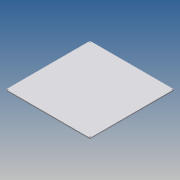
# Autodesk Inventor part: Aluplatte_5mm
Saved by Autodesk Inventor 2015 SP1 (Build 190203100, 203)
## iProperties
Created: 2015-03-05
Part Number: Aluplatte_5mm
Material: Aluminium 6061
Document SubType Name: Modeling
Designer: Marc
Mass: 1652.69 g
Surface Area: 2521.57 cm^2
Volume: 612.107 cm^3
Density: 2.7 g/cm^3
Appearance: Aluminium - flach
Author: Marc
Autodesk Inventor part; units mm, degrees
ref_plane "YZ Plane" through (0, 0, 0) normal (1, 0, 0) x (0, 1, 0)
ref_plane "XZ Plane" through (0, 0, 0) normal (0, 1, 0) x (-1, 0, 0)
ref_plane "XY Plane" through (0, 0, 0) normal (0, 0, 1) x (1, 0, 0)
sketch "Skizze1" plane through (0, 0, 0) normal (0, 0, 1) x (1, 0, 0)
  line L0 (0, -266) -> (0, 266) projected
  line L1 (-266, 0) -> (266, 0) projected
  line L2 (-190, -190) -> (190, -190)
  line L3 (190, -190) -> (190, 190)
  line L4 (190, 190) -> (-190, 190)
  line L5 (-190, 190) -> (-190, -190)
  line L6 (-190, -190) -> (190, 190) construction
  line L7 (190, -190) -> (-190, 190) construction
  point P0 (0, 0)
  dimension "d0" = 380
  dimension "d1" = 380
  constraints: 12 end point, 2 midpoint, 2 parallel, 1 horizontal, 1 perpendicular
  measures "d0" distance of L4.end L3.end
  measures "d1" distance of L3.end L2.end
extrude "Extrusion1" add sketch "Skizze1" along normal blind 5
sketch "Skizze2" plane through (0, 0, 5) normal (0, 0, 1) x (1, 0, 0)
  line L0 (-190, -190) -> (190, -190) projected
  line L1 (190, -190) -> (190, 190) projected
  line L2 (190, 190) -> (-190, 190) projected
  line L3 (-190, 190) -> (-190, -190) projected
  circle A0 centre (-186, 186) radius 2.5
  line L4 (0, -280) -> (0, 280) projected
  line L5 (-280, 0) -> (280, 0) projected
  circle A1 centre (186, 186) radius 2.5
  circle A2 centre (-186, -186) radius 2.5
  circle A3 centre (186, -186) radius 2.5
  point P0 (0, 0)
  dimension "d4" = 5
  dimension "d5" = 4
  dimension "d6" = 4
  constraints: 4 centre point, 3 symmetric about line, 3 other
  measures "d4" diameter of A0
  measures "d5" distance from line of L2 A0.centre
  measures "d6" distance from line of L3 A0.centre
extrude "Extrusion2" cut sketch "Skizze2" against normal blind 5 contours A0 | A1 | A2 | A3
